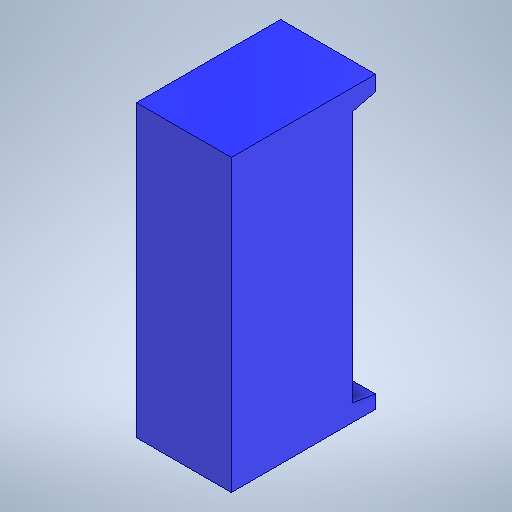
# Autodesk Inventor part: StandLeg
Saved by Autodesk Inventor 2025 (Build 290162010, 162A)
## iProperties
Created: 2024-08-20
Part Number: StandLeg
Material: Generic
Document SubType Name: Modeling
Designer: max_d
Density: 1 g/cm^3
Appearance: Default
Author: max_d
Autodesk Inventor part; units mm, degrees
ref_plane "YZ Plane" through (0, 0, 0) normal (1, 0, 0) x (0, 1, 0)
ref_plane "XZ Plane" through (0, 0, 0) normal (0, 1, 0) x (-1, 0, 0)
ref_plane "XY Plane" through (0, 0, 0) normal (0, 0, 1) x (1, 0, 0)
sketch "Sketch2" plane through (0, 0, 0) normal (1, 0, 0) x (0, 1, 0)
  line L0 (0, 0) -> (765, 0)
  line L1 (765, 0) -> (765, -380)
  line L2 (0, -380) -> (0, 0)
  line L3 (710, -320) -> (45, -320)
  line L4 (0, -380) -> (35, -380)
  line L5 (765, -380) -> (725, -380)
  line L6 (725, -380) -> (710, -320)
  line L7 (45, -320) -> (35, -380)
  dimension "d3" = 380
  dimension "d4" = 320
  dimension "d5" = 35
  dimension "d6" = 40
  dimension "d7" = 765
  dimension "d8" = 55
  dimension "d9" = 45
  constraints: 16 end point, 3 perpendicular, 2 horizontal, 1 collinear, 1 parallel
  measures "d3" distance of L0.end L1.end
  measures "d4" distance between parallel lines of L0 L3
  measures "d5" distance of L2.start L4.end
  measures "d6" distance of L1.end L5.end
  measures "d7" distance of L0.start L0.end
  measures "d8" distance from line of L1 L3.start
  measures "d9" distance from line of L2 L3.end
extrude "Extrusion1" add sketch "Sketch2" along normal blind 250
body "Solid1"
